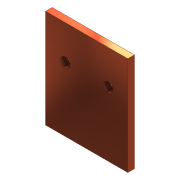
# Autodesk Inventor part: Placa PCB 1,5 x 1,5 cm
Saved by Autodesk Inventor 2020 (Build 240168000, 168)
## iProperties
Created: 2020-08-13
Part Number: Placa PCB 1,5 x 1,5 cm
Material: Generic
Document SubType Name: Modeling
Designer: Dante
Density: 1 g/cm^3
Appearance: Copper - Polished
Author: Dante
Autodesk Inventor part; units mm, degrees
ref_plane "YZ Plane" through (0, 0, 0) normal (1, 0, 0) x (0, 1, 0)
ref_plane "XZ Plane" through (0, 0, 0) normal (0, 1, 0) x (-1, 0, 0)
ref_plane "XY Plane" through (0, 0, 0) normal (0, 0, 1) x (1, 0, 0)
sketch "Sketch1" plane through (0, 0, 0) normal (0, 0, 1) x (1, 0, 0)
  line L0 (-33.6909, 31.0213) -> (-8.6909, 31.0213)
  line L1 (-8.6909, 31.0213) -> (-8.6909, 1.0213)
  line L2 (-8.6909, 1.0213) -> (-33.6909, 1.0213)
  line L3 (-33.6909, 1.0213) -> (-33.6909, 31.0213)
  circle A0 centre (-27.6909, 20.5213) radius 1.5
  circle A1 centre (-14.6909, 20.5213) radius 1.5
  line L4 (-21.1909, 1.0213) -> (-21.1909, 31.0213)
  line L5 (-33.6909, 16.0213) -> (-8.6909, 16.0213)
  dimension "d0" = 25
  dimension "d1" = 30
  dimension "d4" = 3
  dimension "d5" = 3
  dimension "d6" = 13
  dimension "d7" = 6
  dimension "d8" = 10.5
  constraints: 12 end point, 4 midpoint, 2 centre point, 2 parallel, 1 horizontal, 1 perpendicular
  measures "d0" distance of L1.end L2.end
  measures "d1" distance of L0.end L1.end
  measures "d4" diameter of A0
  measures "d5" diameter of A1
  measures "d6" distance of A1.centre A0.centre
  measures "d7" distance from line of L3 A0.centre
  measures "d8" distance from line of A0.centre L0
extrude "Extrusion1" add sketch "Sketch1" along normal blind 2
equation "\"d4\" = d5"
body "Solid1"
